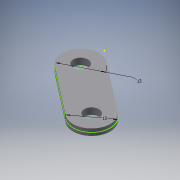
# Autodesk Inventor part: smallthing
Saved by Autodesk Inventor 2018 (Build 220112000, 112)
## iProperties
Created: 2018-12-04
Part Number: smallthing
Material: Generic
Document SubType Name: Modeling
Designer: Jerry
Density: 1 g/cm^3
Appearance: Default
Author: Jerry
Autodesk Inventor part; units mm, degrees
ref_plane "YZ Plane" through (0, 0, 0) normal (1, 0, 0) x (0, 1, 0)
ref_plane "XZ Plane" through (0, 0, 0) normal (0, 1, 0) x (-1, 0, 0)
ref_plane "XY Plane" through (0, 0, 0) normal (0, 0, 1) x (1, 0, 0)
sketch "Sketch1" plane through (0, 0, 0) normal (0, 0, 1) x (1, 0, 0)
  arc A0 (4.9396, -4.0821) -> (-3.0171, -14.3627) centre (0.9613, -9.2224) ccw
  arc A1 (13.9722, -27.5116) -> (21.9289, -17.231) centre (17.9505, -22.3713) ccw
  line L0 (4.9396, -4.0821) -> (21.9289, -17.231)
  line L1 (-3.0171, -14.3627) -> (13.9722, -27.5116)
  point P0 (0, 0)
  dimension "d0" = 13
  dimension "d1" = 13
  constraints: 4 end point, 4 point on circle, 4 tangent, 2 centre point, 2 coincident
  measures "d0" diameter of A0
  measures "d1" diameter of A1
extrude "Extrusion1" add sketch "Sketch1" along normal mid plane 2.2625
hole "Hole1" at (0.9613, -9.2224, 0) at (17.9505, -22.3713, 0) direction (0, 0, 1) diameter 5.159 end through all both
body "Solid1"
